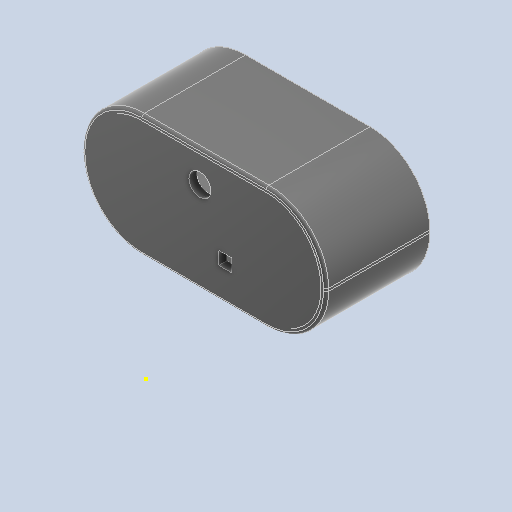
# Autodesk Inventor part: Front
Saved by Autodesk Inventor 2024 (Build 280153000, 153)
## iProperties
Created: 2023-10-04
Part Number: Front
Material: Acetal Resin, Black
Document SubType Name: Modeling
Designer: User Account
Density: 1.425 g/cm^3
Appearance: Smooth - Black
Author: User Account
Autodesk Inventor part; units mm, degrees
ref_plane "YZ Plane" through (0, 0, 0) normal (1, 0, 0) x (0, 1, 0)
ref_plane "XZ Plane" through (0, 0, 0) normal (0, 1, 0) x (-1, 0, 0)
ref_plane "XY Plane" through (0, 0, 0) normal (0, 0, 1) x (1, 0, 0)
sketch "Sketch1" plane through (0, 0, 0) normal (0, 0, 1) x (1, 0, 0)
  line L0 (1.5095, 88.3915) -> (49.5095, 88.3915)
  line L1 (70.5095, 67.3915) -> (70.5095, 66.3915)
  line L2 (49.5095, 45.3915) -> (1.5095, 45.3915)
  line L3 (-19.4905, 66.3915) -> (-19.4905, 67.3915)
  arc A0 (1.5095, 88.3915) -> (-19.4905, 67.3915) centre (1.5095, 67.3915) ccw
  arc A1 (-19.4905, 66.3915) -> (1.5095, 45.3915) centre (1.5095, 66.3915) ccw
  arc A2 (70.5095, 67.3915) -> (49.5095, 88.3915) centre (49.5095, 67.3915) ccw
  arc A3 (49.5095, 45.3915) -> (70.5095, 66.3915) centre (49.5095, 66.3915) ccw
  line L4 (49.5095, 90.3915) -> (1.5095, 90.3915)
  arc A4 (1.5095, 90.3915) -> (-21.4905, 67.3915) centre (1.5095, 67.3915) ccw
  line L5 (-21.4905, 67.3915) -> (-21.4905, 66.3915)
  arc A5 (-21.4905, 66.3915) -> (1.5095, 43.3915) centre (1.5095, 66.3915) ccw
  line L6 (1.5095, 43.3915) -> (49.5095, 43.3915)
  arc A6 (49.5095, 43.3915) -> (72.5095, 66.3915) centre (49.5095, 66.3915) ccw
  line L7 (72.5095, 66.3915) -> (72.5095, 67.3915)
  arc A7 (72.5095, 67.3915) -> (49.5095, 90.3915) centre (49.5095, 67.3915) ccw
  line L8 (1.5095, 45.3915) -> (49.5095, 45.3915)
  line L9 (49.5095, 45.3915) -> (49.5095, 88.3915)
  line L10 (49.5095, 88.3915) -> (1.5095, 88.3915)
  line L11 (1.5095, 88.3915) -> (1.5095, 45.3915)
  point P0 (0, 0)
  point P1 (-19.4905, 88.3915)
  point P2 (70.5095, 45.3915)
  point P3 (70.5095, 88.3915)
  point P4 (-19.4905, 66.8915)
  dimension "d0" = 90
  dimension "d1" = 43
  dimension "d2" = 21
  dimension "d3" = 21
  dimension "d6" = 2
  dimension "d36" = 48
  constraints: 24 end point, 16 point on circle, 8 centre point, 8 tangent, 6 parallel, 6 point on line, 3 perpendicular, 2 equal radius, 2 horizontal, 1 midpoint, 7 other
  measures "d0" distance of point (-19.49, 88.392) point (70.51, 88.392)
  measures "d1" distance of point (70.51, 88.392) point (70.51, 45.392)
  measures "d2" radius of A0
  measures "d3" radius of A1
  measures "d6" distance between parallel lines of L0 L4
  measures "d36" distance of L0.end L0.start
extrude "Extrusion2" add sketch "Sketch1" along normal blind 3 contours L11 A1 L3 A0 | L0 L9 L2 L11 | A2 L1 A3 L9
sketch "Sketch5" plane through (0, 0, 3) normal (0, 0, 1) x (1, 0, 0)
  line L0 (1.5145, 88.3941) -> (49.5145, 88.3941)
  line L1 (70.5145, 67.3941) -> (70.5145, 66.3941)
  line L2 (49.5145, 45.3941) -> (1.5145, 45.3941)
  line L3 (-19.4855, 66.3941) -> (-19.4855, 67.3941)
  arc A0 (1.5145, 88.3941) -> (-19.4855, 67.3941) centre (1.5145, 67.3941) ccw
  arc A1 (-19.4855, 66.3941) -> (1.5145, 45.3941) centre (1.5145, 66.3941) ccw
  arc A2 (70.5145, 67.3941) -> (49.5145, 88.3941) centre (49.5145, 67.3941) ccw
  arc A3 (49.5145, 45.3941) -> (70.5145, 66.3941) centre (49.5145, 66.3941) ccw
  line L4 (49.5145, 90.3941) -> (1.5145, 90.3941)
  arc A4 (1.5145, 90.3941) -> (-21.4855, 67.3941) centre (1.5145, 67.3941) ccw
  line L5 (-21.4855, 67.3941) -> (-21.4855, 66.3941)
  arc A5 (-21.4855, 66.3941) -> (1.5145, 43.3941) centre (1.5145, 66.3941) ccw
  line L6 (1.5145, 43.3941) -> (49.5145, 43.3941)
  arc A6 (49.5145, 43.3941) -> (72.5145, 66.3941) centre (49.5145, 66.3941) ccw
  line L7 (72.5145, 66.3941) -> (72.5145, 67.3941)
  arc A7 (72.5145, 67.3941) -> (49.5145, 90.3941) centre (49.5145, 67.3941) ccw
  circle A8 centre (23.6625, 78.0591) radius 2.25
  line L8 (10.0145, 58.4841) -> (13.8145, 58.4841)
  line L9 (13.8145, 58.4841) -> (13.8145, 54.6841)
  line L10 (13.8145, 54.6841) -> (10.0145, 54.6841)
  line L11 (10.0145, 54.6841) -> (10.0145, 58.4841)
  point P0 (0, 0)
  point P1 (-69.6997, -39.2573)
  point P2 (-19.4855, 88.3941)
  point P3 (70.5145, 45.3941)
  point P4 (70.5145, 88.3941)
  point P5 (-19.4855, 66.8941)
  point P6 (10.0145, 56.5841)
  point P7 (11.9145, 54.6841)
  dimension "d16" = 90
  dimension "d17" = 43
  dimension "d18" = 21
  dimension "d19" = 21
  dimension "d20" = 2
  dimension "d21" = 4.5
  dimension "d22" = 3.8
  dimension "d23" = 29.5
  dimension "d24" = 9.29
  dimension "d25" = 3.8
  dimension "d26" = 43.148
  dimension "d27" = 10.335
  constraints: 24 end point, 16 point on circle, 9 centre point, 8 tangent, 6 parallel, 6 point on line, 3 midpoint, 3 perpendicular, 2 equal radius, 2 horizontal, 7 other
  measures "d16" distance of point (-19.485, 88.394) point (70.515, 88.394)
  measures "d17" distance of point (70.515, 88.394) point (70.515, 45.394)
  measures "d18" radius of A0
  measures "d19" radius of A1
  measures "d20" distance between parallel lines of L0 L4
  measures "d21" diameter of A8
  measures "d22" distance of L8.end L9.end
  measures "d23" horizontal distance of point (-19.485, 66.894) point (10.015, 56.584)
  measures "d24" distance from line of L2 point (11.915, 54.684)
  measures "d25" distance of L8.start L8.end
  measures "d26" horizontal distance of point (-19.485, 66.894) A8.centre
  measures "d27" distance from line of L0 A8.centre
extrude "Extrusion3" add sketch "Sketch5" against normal blind 40 contours A7 L7 A6 L6 A5 L5 A4 L4
fillet "Fillet1" radius 1 8 edges at (-21.4855, 66.8941, 3) (-14.7489, 50.1306, 3) (25.5145, 43.3941, 3) (65.778, 50.1306, 3) (72.5145, 66.8941, 3) (65.778, 83.6576, 3) (25.5145, 90.3941, 3) (-14.7489, 83.6576, 3)
sketch "Sketch7" plane through (0, 0, 3) normal (0, 0, 1) x (1, 0, 0)
  circle A0 centre (23.877, 78.2199) radius 0.1744
  circle A1 centre (23.877, 78.2199) radius 4.25
  line L0 (31.6393, 59.8664) -> (31.2393, 59.8664)
  line L1 (36.1393, 54.9164) -> (35.7393, 54.9164)
  line L2 (31.2393, 59.8664) -> (36.1393, 59.8664)
  line L3 (36.1393, 59.8664) -> (36.1393, 54.9164)
  line L4 (36.1393, 54.9164) -> (31.2393, 54.9164)
  line L5 (31.2393, 54.9164) -> (31.2393, 59.8664)
  line L6 (-2.1134, 89.7222) -> (57.8866, 89.7222)
  line L7 (57.8866, 89.7222) -> (57.8866, 49.7222)
  line L8 (57.8866, 49.7222) -> (-2.1134, 49.7222)
  line L9 (-2.1134, 49.7222) -> (-2.1134, 89.7222)
  point P0 (0, 0)
  point P1 (-83.2087, 35.9088)
  dimension "d40" = 8.5
  dimension "d41" = 60
  dimension "d42" = 40
  constraints: 20 end point, 4 parallel, 2 centre point, 2 horizontal, 2 perpendicular, 1 coincident
  measures "d40" diameter of A1
  measures "d41" distance of L7.end L8.end
  measures "d42" distance of L8.end L6.start
extrude "Extrusion5" cut sketch "Sketch7" against normal blind 10 contours A0 | A1 | L2 L3 L1 L4 L5 L0
sketch "Sketch8" plane through (0, 0, 0) normal (0, 0, -1) x (-1, 0, 0)
  point P0 (0, 0)
body "Solid2"
